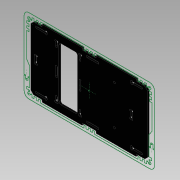
# Autodesk Inventor part: AK-C-C39-Main-Board
Saved by Autodesk Inventor 2016 (Build 200138000, 138)
## iProperties
Created: 2016-04-01
Part Number: AK-C-C39-Main-Board
Material: Generic
Document SubType Name: Modeling
Designer: admin
Density: 1 g/cm^3
Appearance: Smooth - Black
Mass: 8.70772 g
Surface Area: 121.49 cm^2
Volume: 8.70772 cm^3
Author: admin
Autodesk Inventor part; units mm, degrees
ref_plane "YZ Plane" through (0, 0, 0) normal (1, 0, 0) x (0, 1, 0)
ref_plane "XZ Plane" through (0, 0, 0) normal (0, 1, 0) x (-1, 0, 0)
ref_plane "XY Plane" through (0, 0, 0) normal (0, 0, 1) x (1, 0, 0)
derived "SZOMK-AK-C-C39.ipt"
sketch "Sketch1" plane through (0, 0, 0) normal (0, 1, 0) x (-1, 0, 0)
  arc A0 (55.5973, 28.6788) -> (54.2538, 30.0223) centre (55.5, 29.925) ccw
  arc A1 (-54.2538, 30.0223) -> (-55.5973, 28.6788) centre (-55.5, 29.925) ccw
  arc A2 (54.2538, -30.0223) -> (55.5973, -28.6788) centre (55.5, -29.925) ccw
  arc A3 (-55.5973, -28.6788) -> (-54.2538, -30.0223) centre (-55.5, -29.925) ccw
  line L0 (55.5, 34.425) -> (-55.5, 34.425)
  line L1 (55.5, -34.425) -> (-55.5, -34.425)
  line L2 (9.5866, 0) -> (-6.7847, 0) construction
  line L3 (0, -6.6233) -> (0, 6.4737) construction
  arc A4 (55.5, -34.425) -> (60, -29.925) centre (55.5, -29.925) ccw
  arc A5 (60, 29.925) -> (55.5, 34.425) centre (55.5, 29.925) ccw
  arc A6 (-55.5, 34.425) -> (-60, 29.925) centre (-55.5, 29.925) ccw
  arc A7 (-60, -29.925) -> (-55.5, -34.425) centre (-55.5, -29.925) ccw
  line L4 (57.5, 27.225) -> (57.5, 25.225)
  line L5 (57.5, 25.225) -> (55.5, 25.225)
  line L6 (55.5, 25.225) -> (55.5, 23.225)
  line L7 (55.5, 23.225) -> (57.5, 23.225)
  line L8 (57.5, 23.225) -> (57.5, 21.225)
  line L9 (57.5, 21.225) -> (55.5, 21.225)
  line L10 (55.5, 21.225) -> (55.5, 19.225)
  line L11 (55.5, 19.225) -> (57.8, 19.225)
  line L12 (57.8, 19.225) -> (57.8, -3.3607)
  line L13 (-57.5, 27.225) -> (-57.5, 25.225)
  line L14 (-57.5, 25.225) -> (-55.5, 25.225)
  line L15 (-55.5, 25.225) -> (-55.5, 23.225)
  line L16 (-55.5, 23.225) -> (-57.5, 23.225)
  line L17 (-57.5, 23.225) -> (-57.5, 21.225)
  line L18 (-57.5, 21.225) -> (-55.5, 21.225)
  line L19 (-55.5, 21.225) -> (-55.5, 19.225)
  line L20 (-55.5, 19.225) -> (-57.8, 19.225)
  line L21 (-57.8, 19.225) -> (-57.8, -3.3607)
  line L22 (57.5, 27.225) -> (55.3506, 27.225)
  line L23 (52.8, 29.7756) -> (52.8, 31.925)
  line L24 (52.8, 31.925) -> (50.8, 31.925)
  line L25 (50.8, 31.925) -> (50.8, 29.925)
  line L26 (50.8, 29.925) -> (48.8, 29.925)
  line L27 (48.8, 29.925) -> (48.8, 31.925)
  line L28 (48.8, 31.925) -> (46.8, 31.925)
  line L29 (46.8, 31.925) -> (46.8, 29.925)
  line L30 (46.8, 29.925) -> (44.8, 29.925)
  line L31 (44.8, 29.925) -> (44.8, 32.325)
  line L32 (44.8, 32.325) -> (5, 32.325)
  line L33 (5, 32.325) -> (5, 29.925)
  line L34 (5, 29.925) -> (3, 29.925)
  line L35 (3, 29.925) -> (3, 31.925)
  line L36 (3, 31.925) -> (1, 31.925)
  line L37 (1, 31.925) -> (1, 29.925)
  line L38 (1, 29.925) -> (-1, 29.925)
  line L39 (-1, 29.925) -> (-1, 31.925)
  line L40 (-1, 31.925) -> (-3, 31.925)
  line L41 (-3, 31.925) -> (-3, 29.925)
  line L42 (-3, 29.925) -> (-5, 29.925)
  line L43 (-5, 29.925) -> (-5, 32.325)
  line L44 (-5, 32.325) -> (-44.8, 32.325)
  line L45 (-44.8, 32.325) -> (-44.8, 29.925)
  line L46 (-44.8, 29.925) -> (-46.8, 29.925)
  line L47 (-46.8, 29.925) -> (-46.8, 31.925)
  line L48 (-46.8, 31.925) -> (-48.8, 31.925)
  line L49 (-48.8, 31.925) -> (-48.8, 29.925)
  line L50 (-48.8, 29.925) -> (-50.8, 29.925)
  line L51 (-50.8, 29.925) -> (-50.8, 31.925)
  line L52 (-50.8, 31.925) -> (-52.8, 31.925)
  line L53 (-52.8, 31.925) -> (-52.8, 29.7756)
  line L54 (-55.3506, 27.225) -> (-57.5, 27.225)
  line L55 (55.5973, 28.6788) -> (54.9971, 28.0786)
  line L56 (54.2538, 30.0223) -> (53.6536, 29.4221)
  line L57 (55.5, 29.925) -> (51.9091, 26.3341) construction
  arc A8 (52.8, 29.7756) -> (53.6536, 29.4221) centre (53.3, 29.7756) ccw
  arc A9 (54.9971, 28.0786) -> (55.3506, 27.225) centre (55.3506, 27.725) ccw
  line L58 (-55.5973, 28.6788) -> (-54.9971, 28.0786)
  line L59 (-54.2538, 30.0223) -> (-53.6536, 29.4221)
  arc A10 (-53.6536, 29.4221) -> (-52.8, 29.7756) centre (-53.3, 29.7756) ccw
  arc A11 (-55.3506, 27.225) -> (-54.9971, 28.0786) centre (-55.3506, 27.725) ccw
  line L60 (57.8, -3.3607) -> (55, -7.6074)
  line L61 (55, -7.6074) -> (55, -16.775)
  arc A12 (56.5, -18.525) -> (58.5, -18.525) centre (57.5, -19.275) ccw
  line L62 (58.5, -18.525) -> (58.5, -16.775)
  line L63 (56.5, -18.525) -> (56.5, -16.775)
  line L64 (55, -16.775) -> (56.5, -16.775)
  line L65 (58.5, -16.775) -> (60, -16.775)
  line L66 (57.5, -16.4962) -> (57.5, -11.7384) construction
  line L67 (-57.8, -3.3607) -> (-55, -7.6074)
  line L68 (-55, -7.6074) -> (-55, -16.775)
  arc A13 (-56.5, -15.025) -> (-58.5, -15.025) centre (-57.5, -14.275) ccw
  line L69 (-58.5, -15.025) -> (-58.5, -16.775)
  line L70 (-56.5, -15.025) -> (-56.5, -16.775)
  line L71 (-55, -16.775) -> (-56.5, -16.775)
  line L72 (-58.5, -16.775) -> (-60, -16.775)
  line L73 (-57.5, -20.9142) -> (-57.5, -16.6435) construction
  line L74 (44.8, -32.325) -> (5, -32.325)
  line L75 (5, -32.325) -> (5, -29.925)
  line L76 (5, -29.925) -> (3, -29.925)
  line L77 (3, -29.925) -> (3, -31.925)
  line L78 (3, -31.925) -> (1, -31.925)
  line L79 (1, -31.925) -> (1, -29.925)
  line L80 (1, -29.925) -> (-1, -29.925)
  line L81 (-1, -29.925) -> (-1, -31.925)
  line L82 (-1, -31.925) -> (-3, -31.925)
  line L83 (-3, -31.925) -> (-3, -29.925)
  line L84 (-3, -29.925) -> (-5, -29.925)
  line L85 (-5, -29.925) -> (-5, -32.325)
  line L86 (-5, -32.325) -> (-44.8, -32.325)
  line L87 (55, -17.425) -> (55, -25.225)
  line L88 (55, -25.225) -> (57.5, -25.225)
  line L89 (57.5, -25.225) -> (57.5, -27.225)
  line L90 (57.5, -27.225) -> (55.3506, -27.225)
  line L91 (52.8, -29.7756) -> (52.8, -31.925)
  line L92 (52.8, -31.925) -> (50.8, -31.925)
  line L93 (50.8, -31.925) -> (50.8, -29.925)
  line L94 (50.8, -29.925) -> (48.8, -29.925)
  line L95 (48.8, -29.925) -> (48.8, -31.925)
  line L96 (48.8, -31.925) -> (46.8, -31.925)
  line L97 (46.8, -31.925) -> (46.8, -29.925)
  line L98 (46.8, -29.925) -> (44.8, -29.925)
  line L99 (44.8, -29.925) -> (44.8, -32.325)
  line L100 (-44.8, -32.325) -> (-44.8, -29.925)
  line L101 (-44.8, -29.925) -> (-46.8, -29.925)
  line L102 (-46.8, -29.925) -> (-46.8, -31.925)
  line L103 (-46.8, -31.925) -> (-48.8, -31.925)
  line L104 (-48.8, -31.925) -> (-48.8, -29.925)
  line L105 (-48.8, -29.925) -> (-50.8, -29.925)
  line L106 (-50.8, -29.925) -> (-50.8, -31.925)
  line L107 (-50.8, -31.925) -> (-52.8, -31.925)
  line L108 (-52.8, -31.925) -> (-52.8, -29.7756)
  line L109 (-55.3506, -27.225) -> (-57.5, -27.225)
  line L110 (-57.5, -27.225) -> (-57.5, -25.225)
  line L111 (-57.5, -25.225) -> (-55, -25.225)
  line L112 (-55, -25.225) -> (-55, -17.425)
  line L113 (54.9971, -28.0786) -> (55.5973, -28.6788)
  line L114 (53.6536, -29.4221) -> (54.2538, -30.0223)
  arc A14 (55.3506, -27.225) -> (54.9971, -28.0786) centre (55.3506, -27.725) ccw
  arc A15 (53.6536, -29.4221) -> (52.8, -29.7756) centre (53.3, -29.7756) ccw
  line L115 (-54.2538, -30.0223) -> (-53.6536, -29.4221)
  line L116 (-55.5973, -28.6788) -> (-54.9971, -28.0786)
  arc A16 (-52.8, -29.7756) -> (-53.6536, -29.4221) centre (-53.3, -29.7756) ccw
  arc A17 (-54.9971, -28.0786) -> (-55.3506, -27.225) centre (-55.3506, -27.725) ccw
  line L117 (55, -17.425) -> (56.5, -17.425)
  line L118 (58.5, -17.425) -> (60, -17.425)
  line L119 (60, -29.925) -> (60, -17.425)
  line L120 (60, -16.775) -> (60, 29.925)
  line L121 (-55, -17.425) -> (-56.5, -17.425)
  line L122 (-56.5, -17.425) -> (-56.5, -16.775)
  line L123 (-58.5, -16.775) -> (-58.5, -17.425)
  line L124 (-58.5, -17.425) -> (-60, -17.425)
  line L125 (-60, -29.925) -> (-60, -17.425)
  line L126 (-60, -16.775) -> (-60, 29.925)
  point P0 (0, 0)
sketch "Sketch2" plane through (0, 0, 0) normal (0, 1, 0) x (-1, 0, 0)
  line L0 (51.25, -29) -> (44.125, -29)
  line L1 (43.25, -29.875) -> (43.25, -31)
  line L2 (43.25, -31) -> (6.5, -31)
  line L3 (6.5, -31) -> (6.5, -29.875)
  line L4 (5.625, -29) -> (-5.625, -29)
  line L5 (-6.5, -29.875) -> (-6.5, -31)
  line L6 (-6.5, -31) -> (-43.25, -31)
  line L7 (-43.25, -31) -> (-43.25, -29.875)
  line L8 (-44.125, -29) -> (-51.25, -29)
  line L9 (-51.25, -29) -> (-53.75, -26.5)
  line L10 (-53.75, -26.5) -> (-53.75, 26.5)
  line L11 (-53.75, 26.5) -> (-51.25, 29)
  line L12 (-51.25, 29) -> (-44.125, 29)
  line L13 (-43.25, 29.875) -> (-43.25, 31)
  line L14 (-43.25, 31) -> (-6.5, 31)
  line L15 (-6.5, 31) -> (-6.5, 29.875)
  line L16 (-5.625, 29) -> (5.625, 29)
  line L17 (6.5, 29.875) -> (6.5, 31)
  line L18 (43.25, 31) -> (43.25, 29.875)
  line L19 (43.25, 31) -> (6.5, 31)
  line L20 (44.125, 29) -> (51.25, 29)
  line L21 (51.25, 29) -> (53.75, 26.5)
  line L22 (53.75, 26.5) -> (53.75, -26.5)
  line L23 (53.75, -26.5) -> (51.25, -29)
  line L24 (44.8, -32.325) -> (5, -32.325) projected
  line L25 (5, -32.325) -> (5, -29.925) projected
  line L26 (5, -29.925) -> (3, -29.925) projected
  line L27 (44.8, -29.925) -> (44.8, -32.325) projected
  line L28 (46.8, -29.925) -> (44.8, -29.925) projected
  line L29 (52.8, -29.7756) -> (52.8, -31.925) projected
  arc A0 (53.6536, -29.4221) -> (52.8, -29.7756) centre (53.3, -29.7756) ccw projected
  arc A1 (55.3506, -27.225) -> (54.9971, -28.0786) centre (55.3506, -27.725) ccw projected
  line L30 (55, -17.425) -> (55, -25.225) projected
  line L31 (0, -6.6233) -> (0, 6.4737) construction
  line L32 (9.5866, 0) -> (-6.7847, 0) construction
  line L33 (57.8, 19.225) -> (57.8, -3.3607) projected
  line L34 (57.8, -3.3607) -> (55, -7.6074) projected
  line L35 (55.5, 19.225) -> (57.8, 19.225) projected
  line L36 (55.5, 29.925) -> (51.9091, 26.3341) construction
  line L37 (25.75, -24.5) -> (12.75, -24.5)
  line L38 (12.75, 24.5) -> (25.75, 24.5)
  line L39 (3.3524, -20) -> (-16.6476, -20) construction
  line L40 (-16.6476, -20) -> (-16.6476, 20) construction
  line L41 (-16.6476, 20) -> (3.3524, 20) construction
  line L42 (3.3524, 20) -> (3.3524, -20) construction
  line L43 (-23.9878, -15) -> (-31.9878, -15) construction
  line L44 (-31.9878, -15) -> (-31.9878, -7) construction
  line L45 (-31.9878, -7) -> (-23.9878, -7) construction
  line L46 (-23.9878, -7) -> (-23.9878, -15) construction
  line L47 (-34.9878, -15) -> (-42.9878, -15) construction
  line L48 (-42.9878, -15) -> (-42.9878, -7) construction
  line L49 (-42.9878, -7) -> (-34.9878, -7) construction
  line L50 (-34.9878, -7) -> (-34.9878, -15) construction
  line L51 (-23.9878, -4) -> (-31.9878, -4) construction
  line L52 (-31.9878, -4) -> (-31.9878, 4) construction
  line L53 (-31.9878, 4) -> (-23.9878, 4) construction
  line L54 (-23.9878, 4) -> (-23.9878, -4) construction
  line L55 (-34.9878, -4) -> (-42.9878, -4) construction
  line L56 (-42.9878, -4) -> (-42.9878, 4) construction
  line L57 (-42.9878, 4) -> (-34.9878, 4) construction
  line L58 (-34.9878, 4) -> (-34.9878, -4) construction
  line L59 (-23.9878, 7) -> (-31.9878, 7) construction
  line L60 (-31.9878, 7) -> (-31.9878, 15) construction
  line L61 (-31.9878, 15) -> (-23.9878, 15) construction
  line L62 (-23.9878, 15) -> (-23.9878, 7) construction
  line L63 (-34.9878, 7) -> (-42.9878, 7) construction
  line L64 (-42.9878, 7) -> (-42.9878, 15) construction
  line L65 (-42.9878, 15) -> (-34.9878, 15) construction
  line L66 (-34.9878, 15) -> (-34.9878, 7) construction
  line L67 (25.75, -22.5) -> (12.75, -22.5) construction
  line L68 (12.75, -22.5) -> (12.75, -9.5) construction
  line L69 (12.75, -9.5) -> (25.75, -9.5) construction
  line L70 (25.75, -9.5) -> (25.75, -22.5) construction
  line L71 (25.75, -6.5) -> (12.75, -6.5) construction
  line L72 (12.75, -6.5) -> (12.75, 6.5) construction
  line L73 (12.75, 6.5) -> (25.75, 6.5) construction
  line L74 (25.75, 6.5) -> (25.75, -6.5) construction
  line L75 (25.75, 9.5) -> (12.75, 9.5) construction
  line L76 (12.75, 9.5) -> (12.75, 22.5) construction
  line L77 (12.75, 22.5) -> (25.75, 22.5) construction
  line L78 (25.75, 22.5) -> (25.75, 9.5) construction
  line L79 (31.9633, -16) -> (17.7262, -16) construction
  line L80 (31.9633, 16) -> (18.8213, 16) construction
  line L81 (19.25, -23.7063) -> (19.25, 24.6931) construction
  arc A2 (10.75, -22.5) -> (12.75, -24.5) centre (12.75, -22.5) ccw
  arc A3 (25.75, -24.5) -> (27.75, -22.5) centre (25.75, -22.5) ccw
  arc A4 (12.75, 24.5) -> (10.75, 22.5) centre (12.75, 22.5) ccw
  arc A5 (27.75, 22.5) -> (25.75, 24.5) centre (25.75, 22.5) ccw
  line L82 (55, -25.225) -> (-54.9956, -25.225) construction
  line L83 (55.5, 25.225) -> (55.5, 23.225) projected
  line L84 (57.5, 25.225) -> (55.5, 25.225) projected
  line L85 (-57.5, 25.225) -> (-55.5, 25.225) projected
  line L86 (-55.5, 25.225) -> (-55.5, 23.225) projected
  line L87 (-57.5, -25.225) -> (-55, -25.225) projected
  line L88 (-55, -25.225) -> (-55, -17.425) projected
  line L89 (55, -25.225) -> (57.5, -25.225) projected
  line L90 (55.5, 25.225) -> (-55.5, 25.225) construction
  line L91 (48.25, -2.5) -> (48.25, 2.5)
  line L92 (50, -2.5) -> (50, 2.5)
  line L93 (50, -4) -> (48.25, -4)
  line L94 (50, 4) -> (48.25, 4)
  arc A6 (50, -4) -> (50, -2.5) centre (50, -3.25) ccw
  arc A7 (48.25, -2.5) -> (48.25, -4) centre (48.25, -3.25) ccw
  arc A8 (50, 2.5) -> (50, 4) centre (50, 3.25) ccw
  arc A9 (48.25, 4) -> (48.25, 2.5) centre (48.25, 3.25) ccw
  line L95 (-37.75, -2.5) -> (-37.75, 2.5)
  line L96 (-39.5, 4) -> (-37.75, 4)
  line L97 (-39.5, 2.5) -> (-39.5, -2.5)
  line L98 (-39.5, -4) -> (-37.75, -4)
  arc A10 (-37.75, -4) -> (-37.75, -2.5) centre (-37.75, -3.25) ccw
  arc A11 (-39.5, -2.5) -> (-39.5, -4) centre (-39.5, -3.25) ccw
  arc A12 (-37.75, 2.5) -> (-37.75, 4) centre (-37.75, 3.25) ccw
  arc A13 (-39.5, 4) -> (-39.5, 2.5) centre (-39.5, 3.25) ccw
  line L99 (48.75, -27) -> (40.5, -27)
  line L100 (38.75, -27) -> (38.75, -25.25)
  line L101 (40.5, -25.25) -> (48.75, -25.25)
  line L102 (1.75, -27) -> (-8.25, -27)
  line L103 (-8.25, -25.25) -> (1.75, -25.25)
  line L104 (-40, -27) -> (-48.25, -27)
  line L105 (-48.25, -25.25) -> (-40, -25.25)
  line L106 (-48.25, 25.25) -> (-40, 25.25)
  line L107 (-40, 27) -> (-48.25, 27)
  line L108 (1.75, 25.25) -> (-8.25, 25.25)
  line L109 (-8.25, 27) -> (1.75, 27)
  line L110 (48.75, 25.25) -> (40.25, 25.25)
  line L111 (38.75, 25.25) -> (38.75, 27)
  line L112 (40.25, 27) -> (48.75, 27)
  arc A14 (38.75, -27) -> (40.5, -27) centre (39.625, -27) ccw
  arc A15 (40.5, -25.25) -> (38.75, -25.25) centre (39.625, -25.25) ccw
  arc A16 (38.75, 25.25) -> (40.25, 25.25) centre (39.5, 25.25) ccw
  arc A17 (40.25, 27) -> (38.75, 27) centre (39.5, 27) ccw
  line L113 (27.75, 22.5) -> (27.75, -22.5)
  line L114 (-34.9878, 7) -> (-42.9878, 15) construction
  line L115 (-31.9878, 7) -> (-23.9878, 15) construction
  line L116 (-31.9878, -7) -> (-23.9878, -15) construction
  line L117 (-34.9878, -7) -> (-42.9878, -15) construction
  line L118 (10.75, 7.999) -> (10.75, 8)
  line L119 (10.75, -22.5) -> (10.75, 22.5)
  arc A18 (48.75, 25.25) -> (48.75, 27) centre (48.75, 26.125) ccw
  arc A19 (-8.25, 27) -> (-8.25, 25.25) centre (-8.25, 26.125) ccw
  arc A20 (-48.25, 27) -> (-48.25, 25.25) centre (-48.25, 26.125) ccw
  arc A21 (48.75, -27) -> (48.75, -25.25) centre (48.75, -26.125) ccw
  arc A22 (-8.25, -25.25) -> (-8.25, -27) centre (-8.25, -26.125) ccw
  arc A23 (-48.25, -25.25) -> (-48.25, -27) centre (-48.25, -26.125) ccw
  line L120 (31, 25) -> (29.25, 25)
  line L121 (31, 23.5) -> (31, 20)
  line L122 (29.25, 20) -> (29.25, 23.5)
  arc A24 (31, 23.5) -> (31, 25) centre (31, 24.25) ccw
  arc A25 (29.25, 25) -> (29.25, 23.5) centre (29.25, 24.25) ccw
  arc A26 (29.25, 20) -> (31, 20) centre (30.125, 20) ccw
  line L123 (29.25, -20) -> (29.25, -23.25)
  line L124 (29.25, -25) -> (31, -25)
  line L125 (31, -23.25) -> (31, -20)
  arc A27 (31, -25) -> (31, -23.25) centre (31, -24.125) ccw
  arc A28 (29.25, -23.25) -> (29.25, -25) centre (29.25, -24.125) ccw
  arc A29 (31, -20) -> (29.25, -20) centre (30.125, -20) ccw
  line L126 (9.25, 25) -> (7.5, 25)
  line L127 (7.5, 23.5) -> (7.5, 20)
  line L128 (9.25, 20) -> (9.25, 23.5)
  line L129 (7.5, -20) -> (7.5, -23.25)
  line L130 (7.5, -25) -> (9.25, -25)
  line L131 (9.25, -23.25) -> (9.25, -20)
  arc A30 (9.25, -20) -> (7.5, -20) centre (8.375, -20) ccw
  arc A31 (9.25, -25) -> (9.25, -23.25) centre (9.25, -24.125) ccw
  arc A32 (7.5, -23.25) -> (7.5, -25) centre (7.5, -24.125) ccw
  arc A33 (7.5, 20) -> (9.25, 20) centre (8.375, 20) ccw
  arc A34 (9.25, 23.5) -> (9.25, 25) centre (9.25, 24.25) ccw
  arc A35 (7.5, 25) -> (7.5, 23.5) centre (7.5, 24.25) ccw
  line L132 (29.25, 4) -> (29.25, -4)
  line L133 (31, -4) -> (31, 4)
  line L134 (7.5, 4) -> (7.5, -4)
  line L135 (9.25, -4) -> (9.25, 4)
  arc A36 (31, 4) -> (29.25, 4) centre (30.125, 4) ccw
  arc A37 (29.25, -4) -> (31, -4) centre (30.125, -4) ccw
  arc A38 (9.25, 4) -> (7.5, 4) centre (8.375, 4) ccw
  arc A39 (7.5, -4) -> (9.25, -4) centre (8.375, -4) ccw
  line L136 (-14.75, 30.3253) -> (-31.75, 30.3253) construction
  line L137 (-31.75, 30.3253) -> (-31.75, 22.4164) construction
  line L138 (-31.75, 22.4164) -> (-14.75, 22.4164) construction
  line L139 (-14.75, 22.4164) -> (-14.75, 30.3253) construction
  line L140 (-23.25, 29.9722) -> (-23.25, 20.9797) construction
  arc A40 (6.5, -29.875) -> (5.625, -29) centre (5.625, -29.875) ccw
  arc A41 (-5.625, -29) -> (-6.5, -29.875) centre (-5.625, -29.875) ccw
  arc A42 (-43.25, -29.875) -> (-44.125, -29) centre (-44.125, -29.875) ccw
  arc A43 (-44.125, 29) -> (-43.25, 29.875) centre (-44.125, 29.875) ccw
  arc A44 (-6.5, 29.875) -> (-5.625, 29) centre (-5.625, 29.875) ccw
  arc A45 (5.625, 29) -> (6.5, 29.875) centre (5.625, 29.875) ccw
  arc A46 (43.25, 29.875) -> (44.125, 29) centre (44.125, 29.875) ccw
  arc A47 (44.125, -29) -> (43.25, -29.875) centre (44.125, -29.875) ccw
  line L141 (57.5, 27.225) -> (57.5, 25.225) projected
  line L142 (-57.5, 27.225) -> (-57.5, 25.225) projected
  arc A48 (1.75, 25.25) -> (1.75, 27) centre (1.75, 26.125) ccw
  arc A49 (1.75, -27) -> (1.75, -25.25) centre (1.75, -26.125) ccw
  arc A50 (-38.25, 27) -> (-40, 27) centre (-39.125, 27) ccw
  arc A51 (-40, 25.25) -> (-38.25, 25.25) centre (-39.125, 25.25) ccw
  line L143 (-38.25, 27) -> (-38.25, 25.25)
  arc A52 (-38.25, -25.25) -> (-40, -25.25) centre (-39.125, -25.25) ccw
  arc A53 (-40, -27) -> (-38.25, -27) centre (-39.125, -27) ccw
  line L144 (-38.25, -25.25) -> (-38.25, -27)
  line L145 (-60, -16.775) -> (-60, 29.925) projected
  point P0 (53.75, -25.225)
  point P1 (25.75, -16)
  point P2 (25.75, 16)
  point P3 (19.25, -22.5)
  point P4 (19.25, -24.5)
  point P5 (27.75, 0)
  point P6 (10.75, 0)
  point P7 (-23.25, 30.3253)
  point P8 (-23.25, 18)
  point P9 (-23.25, -18)
  point P10 (-53.75, -25.225)
  dimension "d10" = 13
  dimension "d14" = 8
  dimension "d15" = 2
  dimension "d16" = 49
  dimension "d26" = 1.5
  dimension "d28" = 1.75
  dimension "d43" = 20
  dimension "d44" = 40
  dimension "d46" = 3
  dimension "d50" = 29
  dimension "d53" = 17
  dimension "d54" = 10
  dimension "d55" = 10
  dimension "d56" = 5
  dimension "d60" = 1.75
  dimension "d61" = 57
  dimension "d68" = 16
  dimension "d69" = 8
  dimension "d70" = 17
  dimension "d73" = 5
  dimension "d75" = 107.5
  dimension "d78" = 1.75
  dimension "d79" = 20
  dimension "d80" = 0.25
  dimension "d81" = 62
  dimension "d83" = 29
  dimension "d86" = 13
  dimension "d88" = 3
  dimension "d89" = 3
  dimension "d90" = 18
  dimension "d99" = 8
  dimension "d101" = 8.75
  dimension "d102" = 9.25
  dimension "d103" = 7.75
  dimension "d104" = 0.5
  dimension "d105" = 20
  dimension "d106" = 8
  dimension "d121" = 37
  dimension "d122" = 10
  dimension "d123" = 30
  dimension "d124" = 10
  dimension "d126" = 3.75
  dimension "d127" = 10.5
  dimension "d128" = 19.5
  dimension "d129" = 17.5
  dimension "d130" = 42.5
  dimension "d131" = 36.75
  constraints: 248 end point, 104 point on circle, 75 tangent, 64 point on line, 52 centre point, 38 equal radius, 36 parallel, 34 perpendicular, 25 horizontal, 15 collinear, 15 equal length, 7 midpoint, 7 vertical, 6 horizontal alignment, 6 vertical alignment, 4 symmetric about line, 19 other
  measures "d10" distance of L67.end L68.end
  measures "d14" distance of L43.start L43.end
  measures "d15" radius of A2
  measures "d16" distance between parallel lines of L38 L37
  measures "d26" diameter of A6
  measures "d28" distance of L93.start L93.end
  measures "d43" distance of L40.end L41.end
  measures "d44" distance of L39.end L40.end
  measures "d46" distance between parallel lines of L66 L60
  measures "d50" distance between parallel lines of L81 L91
  measures "d53" distance between parallel lines of L119 L113
  measures "d54" distance between parallel lines of L122 L81
  measures "d55" distance from line of L111 A18.centre
  measures "d56" distance from line of A26.centre L120
  measures "d60" distance between parallel lines of L97 L95
  measures "d61" distance between parallel lines of L95 L81
  measures "d68" distance between parallel lines of L32 L80
  measures "d69" distance of A37.centre A36.centre
  measures "d70" distance between parallel lines of L137 L139
  measures "d73" distance from line of A18.centre L22
  measures "d75" distance between parallel lines of L10 L22
  measures "d78" distance between parallel lines of L112 L110
  measures "d79" distance from line of A26.centre L32
  measures "d80" distance between parallel lines of L101 L124
  measures "d81" distance between parallel lines of L2 L19
  measures "d83" distance between parallel lines of L0 L32
  measures "d86" distance between parallel lines of L15 L17
  measures "d88" distance between parallel lines of L59 L53
  measures "d89" distance between parallel lines of L51 L45
  measures "d90" distance from line of L32 point (-23.25, 18)
  measures "d99" distance from line of L18 L20.end
  measures "d101" distance from line of L141 A18.centre
  measures "d102" distance from line of L142 A20.centre
  measures "d103" distance between parallel lines of L111 L121
  measures "d104" distance from line of A18.centre L91
  measures "d105" distance between parallel lines of L128 L122
  measures "d106" distance between parallel lines of L93 L94
  measures "d121" distance from line of A48.centre L111
  measures "d122" distance of A19.centre A48.centre
  measures "d123" distance from line of L143 A19.centre
  measures "d124" distance from line of A20.centre L143
  measures "d126" distance between parallel lines of L92 L22
  measures "d127" distance between parallel lines of L1 L22
  measures "d128" distance between parallel lines of L81 L111
  measures "d129" distance from line of A48.centre L81
  measures "d130" distance from line of point (-23.25, 18) L81
  measures "d131" distance between parallel lines of L145 L140
extrude "Extrusion1" add sketch "Sketch2" along normal blind 1.6
hole "Hole1" at (23.25, 0, 18) at (23.25, 0, -18) direction (0, 1, 0) diameter 2 end through all
sketch "Sketch3" plane through (0, 0, 0) normal (0, -1, 0) x (1, 0, 0)
  line L0 (19.5, -26) -> (27, -26)
  line L1 (27, -26) -> (27, -31)
  line L2 (27, -31) -> (19.5, -31)
  line L3 (19.5, -31) -> (19.5, -26)
  circle A0 centre (23.25, 18) radius 1 projected
  line L4 (43.25, 31) -> (6.5, 31) projected
  line L5 (6.5, -31) -> (43.25, -31) projected
  point P0 (0, 0)
  point P1 (23.25, -31)
  dimension "d108" = 5
  dimension "d109" = 7.5
  constraints: 8 end point, 2 parallel, 1 collinear, 1 horizontal, 1 midpoint, 1 perpendicular, 1 vertical alignment
  measures "d108" distance between parallel lines of L2 L0
  measures "d109" distance of L1.end L2.end
extrude "Extrusion2" [suppressed]
sketch "Sketch4" plane through (43.25, 1.6, -31) normal (0, 0, -1) x (-1, 0, 0)
  line L0 (12.25, -1.2) -> (20.75, -1.2)
  line L1 (20.75, -1.2) -> (20.75, -4.2)
  line L2 (20.75, -4.2) -> (12.25, -4.2)
  line L3 (12.25, -4.2) -> (12.25, -1.2)
  line L4 (20.25, -1.6) -> (20.25, -3.9) projected
  line L5 (20.25, -3.9) -> (12.75, -3.9) projected
  line L6 (12.75, -1.6) -> (12.75, -3.9) projected
  point P0 (-6.5, -1.6)
  dimension "d112" = 3
  dimension "d118" = 0.5
  dimension "d119" = 0.3
  dimension "d120" = 0.5
  constraints: 8 end point, 2 parallel, 1 horizontal, 1 perpendicular
  measures "d112" distance between parallel lines of L2 L0
  measures "d118" distance between parallel lines of L1 L4
  measures "d119" distance between parallel lines of L2 L5
  measures "d120" distance between parallel lines of L6 L3
extrude "Extrusion3" [suppressed]
equation "\"d22\" = d20"
equation "\"d24\" = d20"
equation "\"d20\" = 1.6"
body "Solid1"
